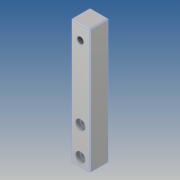
# Autodesk Inventor part: 200-60-DIFFERENTIAL-BAR-01
Saved by Autodesk Inventor 2018.2 (Build 222227000, 227)
## iProperties
Manager: feesmrt
Company: FRANC0R
Created: 2017-12-05
Part Number: 200-60-DIFFERENTIAL-BAR-01
Material: Aluminium 6061
Document SubType Name: Modeling
Designer: feesmrt
Density: 2.7 g/cm^3
Appearance: Aluminium - flach
Project: Rescue Robot
Cost Center: -
Engineer: feesmrt
Authority: feesmrt
Description: Differential Connector Bar
Stock Number: 200-60-DIFFERENTIAL-01
Author: feesmrt
Subject: Rescue Robot
Title: Differential Connector Bar
Revision Number: 1
Autodesk Inventor part; units mm, degrees
ref_plane "YZ Plane" through (0, 0, 0) normal (1, 0, 0) x (0, 1, 0)
ref_plane "XZ Plane" through (0, 0, 0) normal (0, 1, 0) x (-1, 0, 0)
ref_plane "XY Plane" through (0, 0, 0) normal (0, 0, 1) x (1, 0, 0)
sketch "Skizze8" plane through (0, 0, 0) normal (0, 0, 1) x (1, 0, 0)
  line L0 (-10, -10) -> (10, -10)
  line L1 (10, -10) -> (10, 10)
  line L2 (10, 10) -> (-10, 10)
  line L3 (-10, 10) -> (-10, -10)
  line L4 (-10, -10) -> (10, 10) construction
  line L5 (10, -10) -> (-10, 10) construction
  point P0 (0, 0)
  dimension "d49" = 20
  dimension "d50" = 20
  constraints: 12 end point, 2 midpoint, 2 parallel, 1 horizontal, 1 perpendicular
  measures "d49" distance of L0.end L1.end
  measures "d50" distance between parallel lines of L1 L3
extrude "Grundkörper" add sketch "Skizze8" along normal blind 130
sketch "Skizze9" plane through (-10, -10, 0) normal (0, -1, 0) x (1, 0, 0)
  line L0 (10, 156) -> (10, -26) construction
  line L1 (0, 0) -> (20, 0) construction
  point P0 (10, 0)
  point P1 (10, 9)
  point P2 (10, 38.5)
  dimension "d53" = 9
  dimension "d54" = 38.5
  constraints: 2 point on line
  measures "d53" distance from line of L1 point (10, 9)
  measures "d54" distance from line of L1 point (10, 38.5)
hole "DIN7984_M5" at (0, -10, 9) at (0, -10, 38.5) direction (0, 1, 0) diameter 5.5 end through all counterbore diameter 10 counterbore depth 3.9
sketch "Skizze13" plane through (-10, -10, 0) normal (0, -1, 0) x (1, 0, 0)
  line L0 (0, 0) -> (20, 0) projected
  line L1 (10, 156) -> (10, -26) projected
  point P0 (10, 0)
  point P1 (10, 115)
  dimension "d101" = 115
  constraints: 1 point on line
  measures "d101" distance from line of L0 point (10, 115)
hole "M8_Bohrung" at (0, -10, 115) direction (0, 1, 0) diameter 6.647 end through all thread size "M8x1.25" class "6H" standard "ISO Metric profile"
chamfer "Fase_Allgemein" distance 1 angle 45 8 edges at (-10, -10, 65) (0, -10, 130) (10, -10, 65) (-10, 10, 65) (0, 10, 130) (10, 10, 65) (10, 0, 130) (-10, 0, 130)
